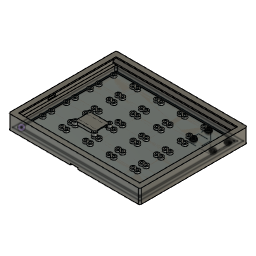
Rpi-LED-Screen v6 (Autodesk Fusion 360 design; units mm, degrees)
Autodesk Fusion 360 part; units mm, degrees
sketch "Sketch1" plane through (0, 0, 0) normal (0, 0, 1) x (1, 0, 0) in component "baseplate"
  line L0 (0, 0) -> (162.5, 0)
  line L1 (162.5, 0) -> (162.5, 130)
  line L2 (162.5, 130) -> (0, 130)
  line L3 (0, 130) -> (0, 0)
  line L4 (-6, -6) -> (168.5, -6)
  line L5 (168.5, -6) -> (168.5, 136)
  line L6 (168.5, 136) -> (-6, 136)
  line L7 (-6, 136) -> (-6, -6)
  line L8 (-2, -2) -> (164.5, -2)
  line L9 (164.5, -2) -> (164.5, 132)
  line L10 (164.5, 132) -> (-2, 132)
  line L11 (-2, 132) -> (-2, -2)
  line L12 (162.5, 130) -> (129.5, 130) construction
  line L13 (129.5, 130) -> (129.5, 97.5) construction
  line L14 (129.5, 97.5) -> (162.5, 97.5) construction
  line L15 (162.5, 97.5) -> (162.5, 130) construction
  line L16 (162.5, 130) -> (160.8, 130) construction
  line L17 (160.8, 130) -> (160.8, 125.5) construction
  line L18 (160.8, 125.5) -> (162.5, 125.5) construction
  line L19 (162.5, 125.5) -> (162.5, 130) construction
  line L20 (160.8, 125.5) -> (159.3, 125.5) construction
  line L21 (159.3, 125.5) -> (159.3, 124) construction
  line L22 (159.3, 124) -> (160.8, 124) construction
  line L23 (160.8, 124) -> (160.8, 125.5) construction
  circle A0 centre (159.3, 124) radius 1.5
  line L24 (162.5, 97.5) -> (129.5, 130) construction
  line L25 (146, 113.75) -> (146, 97.5) construction
  line L26 (129.5, 113.75) -> (146, 113.75) construction
  circle A1 centre (159.3, 124) radius 3.2
  circle A2 centre (159.3, 103.5) radius 3.2
  circle A3 centre (159.3, 103.5) radius 1.5
  circle A4 centre (132.7, 103.5) radius 3.2
  circle A5 centre (132.7, 103.5) radius 1.5
  circle A6 centre (132.7, 124) radius 3.2
  circle A7 centre (132.7, 124) radius 1.5
  dimension "d1" = 162.5
  dimension "d2" = 130
  dimension "d3" = 6
  dimension "d13" = 2
  dimension "d14" = 33
  dimension "d15" = 32.5
  dimension "d16" = 1.7
  dimension "d17" = 4.5
  dimension "d18" = 1.5
  dimension "d19" = 1.5
  dimension "d20" = 3
  dimension "d21" = 1.7
  constraint horizontal L0
  constraint vertical L1
  constraint horizontal L2
  constraint vertical L3
  constraint coincident L0.start L3.end
  constraint horizontal L12
  constraint vertical L13
  constraint horizontal L14
  constraint vertical L15
  constraint horizontal L16
  constraint vertical L17
  constraint horizontal L18
  constraint vertical L19
  constraint horizontal L20
  constraint vertical L21
  constraint horizontal L22
  constraint vertical L23
  constraint coincident L21.end L22.start
  constraint midpoint L24 L25.start
  constraint midpoint L14 L25.end
  constraint midpoint L13 L26.start
  constraint symmetric A0 L26 A3
  constraint symmetric L26 A1 A2
  constraint symmetric A0 L25 A7
  constraint symmetric L25 A1 A6
  constraint symmetric L25 A2 A4
  constraint symmetric L25 A3 A5
  measures "d1" distance of L0.start L0.end
  measures "d2" distance of L0.start L2.end
  measures "d14" distance of L1.end L12.end
  measures "d15" distance of L1.end L14.end
  measures "d16" distance of L1.end L16.end
  measures "d17" distance of L1.end L18.end
  measures "d18" distance of L17.end L20.end
  measures "d19" distance of L17.end L22.end
  measures "d20" diameter of A0
extrude "Extrude1" add sketch "Sketch1" against normal blind 2.4 contours A2 | A1 | L0 L1 L2 L3 | L4 L5 L6 L7 | L8 L9 L10 L11 | A0 | A3 | A4 | A5 | A6 | A7 makes body 1 in component "baseplate"
extrude "Extrude2" add sketch "Sketch1" along normal blind 2.5 contours A2 | A1 | A4 | A6 bodies 1 in component "baseplate"
pattern_linear "R-Pattern1" count 5 spacing 32.5 along (-1, 0, 0) count 4 spacing 32.5 along (0, -1, 0) of "Extrude2" in component "baseplate"
extrude "Extrude3" add sketch "Sketch1" along normal blind 7 contours L4 L5 L6 L7 bodies 1 in component "baseplate"
fillet "Fillet1" radius 5 4 edges at (168.5, 136, 2.3) (-6, 136, 2.3) (168.5, -6, 2.3) (-6, -6, 2.3) on bodies 1 in component "baseplate"
fillet "Fillet1" radius 2 4 edges at (164.5, 132, 3.5) (-2, 132, 3.5) (-2, -2, 3.5) (164.5, -2, 3.5) on bodies 1 in component "baseplate"
fillet "Fillet2" radius 2 8 edges at (-4.5355, -4.5355, -2.4) (-6, 65, -2.4) (-4.5355, 134.5355, -2.4) (81.25, 136, -2.4) (167.0355, 134.5355, -2.4) (168.5, 65, -2.4) (167.0355, -4.5355, -2.4) (81.25, -6, -2.4) on bodies 1 in component "baseplate"
sketch "Sketch1 (2)" plane through (0, 0, 2.5) normal (0, 0, 1) x (-1, 0, 0) in component "PicoAdapter"
  circle A0 centre (-61.8, -103.5) radius 1.5
  arc A1 (-64.75, -102.26) -> (-64.75, -104.74) centre (-67.7, -103.5) ccw
  arc A2 (-64.75, -104.74) -> (-64.75, -102.26) centre (-61.8, -103.5) ccw
  circle A3 centre (-67.7, -103.5) radius 1.5
  circle A4 centre (-35.2, -59) radius 1.5
  circle A5 centre (-61.8, -59) radius 1.5
  circle A6 centre (-61.8, -38.5) radius 1.5
  circle A7 centre (-35.2, -38.5) radius 1.5
  circle A8 centre (-35.2, -59) radius 3
  circle A9 centre (-61.8, -59) radius 3
  circle A10 centre (-61.8, -38.5) radius 3
  circle A11 centre (-35.2, -38.5) radius 3
  line L0 (-35.2, -59) -> (-61.8, -59)
  line L1 (-61.8, -59) -> (-61.8, -38.5)
  line L2 (-61.8, -38.5) -> (-35.2, -38.5)
  line L3 (-35.2, -38.5) -> (-35.2, -59)
  dimension "d38" = 1.5
  dimension "d39" = 1.5
  dimension "d40" = 1.5
  dimension "d41" = 1.5
  constraint horizontal L0
  constraint vertical L1
  constraint horizontal L2
  constraint vertical L3
  constraint coincident A6.centre A10.centre
  constraint coincident A4.centre A8.centre
  measures "d38" distance of A4
  measures "d39" distance of A5
  measures "d40" distance of A6
  measures "d41" distance of A7
extrude "Extrude1'" add sketch "Sketch1 (2)" along normal blind 4 separate body contours A4 A8 L0 L3 | A4 A8 L0 L3 | A8 A9 A10 A11 L0 L1 L2 L3 | A7 A11 L2 L3 | A7 A11 L2 L3 | A5 A9 L0 L1 | A5 A9 L0 L1 | A6 A10 L1 L2 | A6 A10 L1 L2 makes body 2 in component "PicoAdapter"
sketch "Sketch2" plane through (0, 0, 2.5) normal (0, 0, -1) x (1, 0, 0) in component "PicoAdapter"
  circle A0 centre (35.2, -38.5) radius 1.5
  circle A1 centre (61.8, -38.5) radius 1.5
  circle A2 centre (61.8, -59) radius 1.5
  circle A3 centre (35.2, -59) radius 1.5
  arc A4 (35.2, -56) -> (38.2, -59) centre (35.2, -59) ccw
  line L0 (38.2, -59) -> (58.8, -59)
  arc A5 (58.8, -59) -> (61.8, -56) centre (61.8, -59) ccw
  line L1 (61.8, -56) -> (61.8, -41.5)
  arc A6 (61.8, -41.5) -> (58.8, -38.5) centre (61.8, -38.5) ccw
  line L2 (58.8, -38.5) -> (38.2, -38.5)
  arc A7 (38.2, -38.5) -> (35.2, -41.5) centre (35.2, -38.5) ccw
  line L3 (35.2, -41.5) -> (35.2, -56)
  line L4 (35.2, -48.75) -> (61.8, -48.75) construction
  line L5 (35.2, -48.75) -> (61.8, -48.75) construction
  line L6 (61.8, -48.75) -> (61.8, -54.75)
  line L7 (61.8, -54.75) -> (35.2, -54.75)
  line L8 (35.2, -54.75) -> (35.2, -48.75)
  line L9 (61.8, -48.75) -> (35.2, -48.75)
  line L10 (35.2, -48.75) -> (35.2, -42.75)
  line L11 (35.2, -42.75) -> (61.8, -42.75)
  line L12 (61.8, -42.75) -> (61.8, -48.75)
  dimension "d44" = 6
  dimension "d45" = 6
  constraint midpoint L3 L4.start
  constraint midpoint L1 L4.end
  constraint horizontal L5
  constraint vertical L6
  constraint horizontal L7
  constraint vertical L8
  constraint coincident L1 L6.end
  constraint horizontal L9
  constraint vertical L10
  constraint horizontal L11
  constraint vertical L12
  constraint coincident L3 L10.end
  measures "d44" distance of L4.start L7.end
  measures "d45" distance of L4.end L11.end
extrude "Extrude2'" cut sketch "Sketch2" against normal blind 3 contours L1 L3 L6 L7 L8 L9 | L1 L3 L9 L10 L11 L12 bodies 2 in component "PicoAdapter"
ref_plane "WorkPlane1" through (81.25, 65, 17) normal (0, 0, 1) x (1, 0, 0) in component "topcover"
sketch "Sketch1 (3)" plane through (81.25, 65, 17) normal (0, 0, 1) x (1, 0, 0) in component "topcover"
  line L0 (87.25, 71) -> (-87.25, 71)
  line L1 (-87.25, 71) -> (-87.25, -71)
  line L2 (87.25, -71) -> (87.25, 71)
  line L3 (-87.25, -71) -> (87.25, -71)
  line L4 (-87.75, -71.5) -> (87.75, -71.5)
  line L5 (87.75, -71.5) -> (87.75, 71.5)
  line L6 (87.75, 71.5) -> (-87.75, 71.5)
  line L7 (-87.75, 71.5) -> (-87.75, -71.5)
  line L8 (-83.25, 67) -> (-83.25, -67)
  line L9 (83.25, 67) -> (-83.25, 67)
  line L10 (-83.25, -67) -> (83.25, -67)
  line L11 (83.25, -67) -> (83.25, 67)
  line L12 (90.15, -73.9) -> (90.15, 73.9)
  line L13 (90.15, 73.9) -> (-90.15, 73.9)
  line L14 (-90.15, 73.9) -> (-90.15, -73.9)
  line L15 (-90.15, -73.9) -> (90.15, -73.9)
  dimension "d49" = 0.5
  dimension "d50" = 2.9
extrude "Extrude1''" add sketch "Sketch1 (3)" against normal up to surface (19.4 mm away) separate body contours L12 L13 L14 L15 makes body 3 in component "topcover"
extrude "Extrude2''" add sketch "Sketch1 (3)" against normal blind 1.6 contours L0 L1 L2 L3 | L4 L5 L6 L7 bodies 3 in component "topcover"
sketch "Sketch2 (2)" plane through (-8.9, 0, 0) normal (-1, 0, 0) x (0, -1, 0) in component "topcover"
  line L0 (-138.9, -2.4) -> (8.9, -2.4)
  line L1 (8.9, -2.4) -> (8.9, 17)
  line L2 (8.9, 17) -> (-138.9, 17)
  line L3 (-138.9, 17) -> (-138.9, -2.4)
  line L4 (6, 17) -> (6, -2.4) construction
  line L5 (6, -2.4) -> (6, 7.6) construction
  line L6 (6, 7.6) -> (-43, 7.6) construction
  line L7 (-43, 7.6) -> (-53, 7.6) construction
  line L8 (-43, 7.6) -> (-53, 7.6)
  line L9 (-53, 7.6) -> (-53, 12.6)
  line L10 (-53, 12.6) -> (-43, 12.6)
  line L11 (-43, 12.6) -> (-43, 7.6)
  point P0 (6, 17)
  dimension "d55" = 10
  dimension "d56" = 49
  dimension "d57" = 10
  dimension "d58" = 10
  dimension "d59" = 5
  constraint coincident P0 L4.start
  constraint coincident L0 L4.end
  constraint perpendicular L0 L4
  constraint perpendicular L0 L5
  constraint horizontal L6
  constraint horizontal L7
  constraint horizontal L8
  constraint vertical L9
  constraint horizontal L10
  constraint vertical L11
  measures "d55" distance of L4.end L5.end
  measures "d56" distance of L5.end L6.end
  measures "d57" distance of L6.end L7.end
  measures "d58" distance of L6.end L7.end
  measures "d59" distance of L6.end L10.end
extrude "Extrude3'" cut sketch "Sketch2 (2)" against normal blind 2.4 contours L8 L9 L10 L11 bodies 3 in component "topcover"
sketch "Sketch3" plane through (0, 0, 7) normal (0, 0, 1) x (-1, 0, 0) in component "topcover"
  line L0 (2, 0) -> (2, -130)
  arc A0 (0, -132) -> (2, -130) centre (0, -130) ccw
  line L1 (0, -132) -> (-162.5, -132)
  arc A1 (-164.5, -130) -> (-162.5, -132) centre (-162.5, -130) ccw
  line L2 (-164.5, -130) -> (-164.5, 0)
  arc A2 (-162.5, 2) -> (-164.5, 0) centre (-162.5, 0) ccw
  line L3 (-162.5, 2) -> (0, 2)
  arc A3 (2, 0) -> (0, 2) centre (0, 0) ccw
  arc A4 (6, 1) -> (1, 6) centre (1, 1) ccw
  line L4 (1, 6) -> (-163.5, 6)
  arc A5 (-163.5, 6) -> (-168.5, 1) centre (-163.5, 1) ccw
  line L5 (-168.5, 1) -> (-168.5, -131)
  arc A6 (-168.5, -131) -> (-163.5, -136) centre (-163.5, -131) ccw
  line L6 (-163.5, -136) -> (1, -136)
  arc A7 (1, -136) -> (6, -131) centre (1, -131) ccw
  line L7 (6, -131) -> (6, 1)
  line L8 (6.5, -136.5) -> (-169, -136.5)
  line L9 (-169, -136.5) -> (-169, -132)
  line L10 (-169, -132) -> (6.5, -132)
  line L11 (6.5, -132) -> (6.5, -136.5)
  line L12 (-169, 6.5) -> (6.5, 6.5)
  line L13 (6.5, 6.5) -> (6.5, 2)
  line L14 (6.5, 2) -> (-169, 2)
  line L15 (-169, 2) -> (-169, 6.5)
  constraint horizontal L8
  constraint vertical L9
  constraint horizontal L10
  constraint vertical L11
  constraint horizontal L12
  constraint vertical L13
  constraint horizontal L14
  constraint vertical L15
extrude "Extrude4" add sketch "Sketch3" along normal blind 1.6 contours L3 A4 L4 A5 L14 | L1 A6 L6 A7 L10 | A4 L4 A5 L12 L13 L14 L15 | A6 L6 A7 L8 L9 L10 L11 bodies 3 in component "topcover"
draft "Draft1" angle 45 neutral plane through (162.5, -2, 7) pull (0, 1, 0) 1 faces at (54.1667, -5, 8.6) on bodies 3 in component "topcover"
draft "Draft2" angle 45 neutral plane through (168.399, 132, 7) pull (0, -1, 0) 1 faces at (54.1667, 135, 8.6) on bodies 3 in component "topcover"
fillet "Fillet1'" radius 2 4 edges at (171.4, -8.9, 7.3) (171.4, 138.9, 7.3) (-8.9, -8.9, 7.3) (-8.9, 138.9, 7.3) on bodies 3 in component "topcover"
sketch "Sketch4" plane through (0, 0, -2.4) normal (0, 0, -1) x (1, 0, 0) in component "topcover"
  arc A0 (-8.9, -136.9) -> (-6.9, -138.9) centre (-6.9, -136.9) ccw
  line L0 (-6.9, -138.9) -> (169.4, -138.9)
  arc A1 (169.4, -138.9) -> (171.4, -136.9) centre (169.4, -136.9) ccw
  line L1 (171.4, -136.9) -> (171.4, 6.9)
  arc A2 (171.4, 6.9) -> (169.4, 8.9) centre (169.4, 6.9) ccw
  line L2 (169.4, 8.9) -> (-6.9, 8.9)
  arc A3 (-6.9, 8.9) -> (-8.9, 6.9) centre (-6.9, 6.9) ccw
  line L3 (-8.9, 6.9) -> (-8.9, -136.9)
  line L4 (169, -136.5) -> (-6.5, -136.5)
  line L5 (-6.5, -136.5) -> (-6.5, 6.5)
  line L6 (-6.5, 6.5) -> (169, 6.5)
  line L7 (169, 6.5) -> (169, -136.5)
  line L8 (81.25, 6.5) -> (81.25, 8.9) construction
  line L9 (81.25, 6.5) -> (86.25, 6.5)
  line L10 (86.25, 6.5) -> (86.25, 8.9)
  line L11 (86.25, 8.9) -> (81.25, 8.9)
  line L12 (81.25, 8.9) -> (81.25, 6.5)
  line L13 (81.25, 6.5) -> (76.25, 6.5)
  line L14 (76.25, 6.5) -> (76.25, 8.9)
  line L15 (76.25, 8.9) -> (81.25, 8.9)
  line L16 (81.25, 8.9) -> (81.25, 6.5)
  dimension "d70" = 5
  constraint midpoint L6 L8.start
  constraint midpoint L2 L8.end
  constraint horizontal L9
  constraint vertical L10
  constraint horizontal L11
  constraint vertical L12
  constraint horizontal L13
  constraint vertical L14
  constraint horizontal L15
  constraint vertical L16
  constraint coincident L2 L14.end
  measures "d70" distance of L8.start L9.end
extrude "Extrude5" cut sketch "Sketch4" against normal blind 2 contours L2 L6 L12 L13 L14 L15 L16 | L2 L6 L9 L10 L11 L12 L16 bodies 3 in component "topcover"
component "baseplate" placed x (1, 0, 0) y (0, 1, 0) z (0, 0, 1) at (0, 0, 0)
component "PicoAdapter" placed x (1, 0, 0) y (0, 1, 0) z (0, 0, 1) at (0, 0, 0)
component "topcover" placed x (1, 0, 0) y (0, 1, 0) z (0, 0, 1) at (0, 0, 0)
equation "d1 = ( 32.5 * 5 ) * 1 mm"
equation "d2 = ( 32.5 * 4 ) * 1 mm"
equation "d28 = ( 32.5 * 4 ) * 1 mm"
equation "d29 = ( 32.5 * 3 ) * 1 mm"
